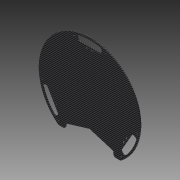
# Autodesk Inventor part: Bottom Plate
Saved by Autodesk Inventor 2015 (Build 190159000, 159)
## iProperties
Created: 2016-08-08
Part Number: Bottom Plate
Material: Generic
Document SubType Name: Modeling
Designer: James Yelland
Density: 1 g/cm^3
Appearance: Default
Author: James Yelland
Autodesk Inventor part; units mm, degrees
ref_plane "YZ Plane" through (0, 0, 0) normal (1, 0, 0) x (0, 1, 0)
ref_plane "XZ Plane" through (0, 0, 0) normal (0, 1, 0) x (-1, 0, 0)
ref_plane "XY Plane" through (0, 0, 0) normal (0, 0, 1) x (1, 0, 0)
sketch "Sketch1" plane through (0, 0, 0) normal (0, 1, 0) x (-1, 0, 0)
  line L0 (-62.9285, -83) -> (-54.3117, -83)
  line L1 (62.9285, -83) -> (54.3117, -83)
  arc A0 (65.4207, -82.1287) -> (-65.4207, -82.1287) centre (0, 0) ccw
  line L2 (-49.3117, -78) -> (-49.3117, -74.4821)
  line L3 (-47.8938, -72.5687) -> (0, -58)
  line L4 (49.3117, -78) -> (49.3117, -74.4821)
  line L5 (47.8938, -72.5687) -> (0, -58)
  arc A1 (49.3117, -78) -> (54.3117, -83) centre (54.3117, -78) ccw
  arc A2 (-54.3117, -83) -> (-49.3117, -78) centre (-54.3117, -78) ccw
  arc A3 (49.3117, -74.4821) -> (47.8938, -72.5687) centre (47.3117, -74.4821) ccw
  arc A4 (-47.8938, -72.5687) -> (-49.3117, -74.4821) centre (-47.3117, -74.4821) ccw
  arc A5 (62.9285, -83) -> (65.4207, -82.1287) centre (62.9285, -79) ccw
  arc A6 (-65.4207, -82.1287) -> (-62.9285, -83) centre (-62.9285, -79) ccw
  line L6 (-76.2102, -44) -> (-65.7102, -62.1865)
  line L7 (-67.1743, -67.6506) -> (-69.6351, -69.0713)
  line L8 (-94.6351, -25.7701) -> (-92.1743, -24.3494)
  line L9 (-86.7102, -25.8135) -> (-76.2102, -44)
  arc A7 (-96.4496, -30.438) -> (-74.5849, -68.3088) centre (0, 0) ccw
  arc A8 (-94.6351, -25.7701) -> (-96.4496, -30.438) centre (-92.6351, -29.2342) ccw
  arc A9 (-86.7102, -25.8135) -> (-92.1743, -24.3494) centre (-90.1743, -27.8135) ccw
  arc A10 (-67.1743, -67.6506) -> (-65.7102, -62.1865) centre (-69.1743, -64.1865) ccw
  arc A11 (-74.5849, -68.3088) -> (-69.6351, -69.0713) centre (-71.6351, -65.6072) ccw
  line L10 (76.2102, -44) -> (86.7102, -25.8135)
  line L11 (92.1743, -24.3494) -> (94.6351, -25.7701)
  line L12 (69.6351, -69.0713) -> (67.1743, -67.6506)
  line L13 (65.7102, -62.1865) -> (76.2102, -44)
  arc A12 (74.5849, -68.3088) -> (96.4496, -30.438) centre (0, 0) ccw
  arc A13 (69.6351, -69.0713) -> (74.5849, -68.3088) centre (71.6351, -65.6072) ccw
  arc A14 (65.7102, -62.1865) -> (67.1743, -67.6506) centre (69.1743, -64.1865) ccw
  arc A15 (92.1743, -24.3494) -> (86.7102, -25.8135) centre (90.1743, -27.8135) ccw
  arc A16 (96.4496, -30.438) -> (94.6351, -25.7701) centre (92.6351, -29.2342) ccw
  line L14 (0, 88) -> (-21, 88)
  line L15 (-25, 92) -> (-25, 94.8414)
  line L16 (25, 94.8414) -> (25, 92)
  line L17 (21, 88) -> (0, 88)
  arc A17 (21.8647, 98.7468) -> (-21.8647, 98.7468) centre (0, 0) ccw
  arc A18 (25, 94.8414) -> (21.8647, 98.7468) centre (21, 94.8414) ccw
  arc A19 (21, 88) -> (25, 92) centre (21, 92) ccw
  arc A20 (-25, 92) -> (-21, 88) centre (-21, 92) ccw
  arc A21 (-21.8647, 98.7468) -> (-25, 94.8414) centre (-21, 94.8414) ccw
  circle A22 centre (-33, 93.4207) radius 1.6
  circle A23 centre (33, 93.4207) radius 1.6
  line L18 (-75.1122, -39.9019) -> (-77.6122, -35.5718)
  line L19 (-77.6122, -35.5718) -> (-75.8801, -34.5718)
  line L20 (-75.8801, -34.5718) -> (-73.3801, -38.9019)
  line L21 (-73.3801, -38.9019) -> (-75.1122, -39.9019)
  line L22 (-72.1122, -45.0981) -> (-69.6122, -49.4282)
  line L23 (-69.6122, -49.4282) -> (-67.8801, -48.4282)
  line L24 (-67.8801, -48.4282) -> (-70.3801, -44.0981)
  line L25 (-70.3801, -44.0981) -> (-72.1122, -45.0981)
  line L26 (72.1122, -45.0981) -> (69.6122, -49.4282)
  line L27 (69.6122, -49.4282) -> (67.8801, -48.4282)
  line L28 (67.8801, -48.4282) -> (70.3801, -44.0981)
  line L29 (70.3801, -44.0981) -> (72.1122, -45.0981)
  line L30 (73.3801, -38.9019) -> (75.1122, -39.9019)
  line L31 (75.8801, -34.5718) -> (73.3801, -38.9019)
  line L32 (77.6122, -35.5718) -> (75.8801, -34.5718)
  line L33 (75.1122, -39.9019) -> (77.6122, -35.5718)
  line L34 (3, 85) -> (8, 85)
  line L35 (8, 85) -> (8, 83)
  line L36 (8, 83) -> (3, 83)
  line L37 (3, 83) -> (3, 85)
  line L38 (-3, 83) -> (-3, 85)
  line L39 (-8, 83) -> (-3, 83)
  line L40 (-8, 85) -> (-8, 83)
  line L41 (-3, 85) -> (-8, 85)
  circle A24 centre (-64.4047, -75.2892) radius 1.6
  circle A25 centre (-97.4047, -18.1315) radius 1.6
  circle A26 centre (97.4047, -18.1315) radius 1.6
  circle A27 centre (64.4047, -75.2892) radius 1.6
  point P0 (64.3117, -83)
  point P1 (-64.3117, -83)
  point P2 (-49.3117, -83)
  point P3 (49.3117, -83)
  point P4 (-49.3117, -73)
  point P5 (49.3117, -73)
  point P6 (-63.7102, -65.6506)
  point P7 (-72.3705, -70.6506)
  point P8 (-97.3705, -27.3494)
  point P9 (88.7102, -22.3494)
  point P10 (97.3705, -27.3494)
  point P11 (-25, 88)
  point P12 (-25, 98)
  dimension "d65" = 360
  dimension "d68" = 3.2
  dimension "d70" = 3.2
  dimension "d79" = 360
  dimension "d83" = 360
  constraints: 84 end point, 50 point on circle, 28 centre point, 20 point on line, 2 perpendicular, 1 coincident, 63 other
  measures "d68" diameter of A22
  measures "d70" diameter of A23
extrude "Extrusion1" add sketch "Sketch1" along normal blind 2
body "Solid1"
